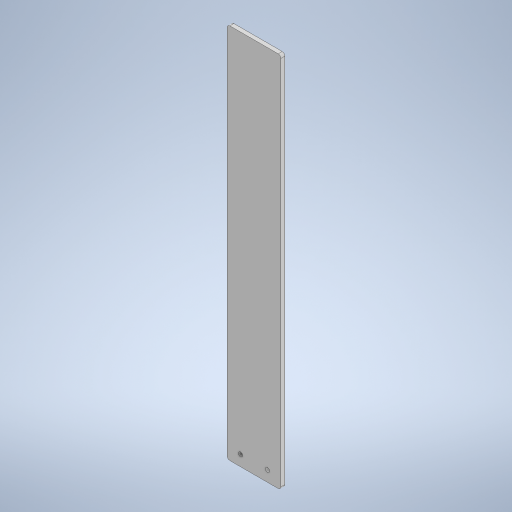
# Autodesk Inventor part: BP_BOX-Support-Bar-Front
Saved by Autodesk Inventor 2024.3 (Build 283343000, 343)
## iProperties
Created: 2025-12-10
Part Number: BP_BOX-Support-Bar-Front
Material: 一般
Document SubType Name: Modeling
Designer: 佐藤智貴
Density: 1 g/cm^3
Appearance: 既定
Author: 佐藤智貴
Autodesk Inventor part; units mm, degrees
ref_plane "YZ Plane" through (0, 0, 0) normal (1, 0, 0) x (0, 1, 0)
ref_plane "XZ Plane" through (0, 0, 0) normal (0, 1, 0) x (-1, 0, 0)
ref_plane "XY Plane" through (0, 0, 0) normal (0, 0, 1) x (1, 0, 0)
sketch "スケッチ1" plane through (0, 0, 0) normal (0, 0, 1) x (1, 0, 0)
  line L0 (0, 0) -> (40, 0)
  line L1 (40, 0) -> (40, 280)
  line L2 (40, 280) -> (0, 280)
  line L3 (0, 280) -> (0, 0)
  dimension "d0" = 40
  dimension "d1" = 280
  constraints: 8 end point, 2 parallel, 1 horizontal, 1 perpendicular
  measures "d0" distance of L1.end L2.end
  measures "d1" distance of L0.end L1.end
extrude "押し出し1" add sketch "スケッチ1" along normal blind 3
sketch "スケッチ2" plane through (0, 0, 3) normal (0, 0, 1) x (1, 0, 0)
  line L0 (0, 280) -> (0, 0) projected
  line L1 (0, 0) -> (40, 0) projected
  point P0 (10, 8)
  point P1 (30, 8)
  point P2 (20, 0)
  dimension "d4" = 20
  dimension "d5" = 10
  dimension "d6" = 8
  constraints: 1 midpoint
  measures "d4" distance of point (30, 8) point (10, 8)
  measures "d5" distance from line of L0 point (10, 8)
  measures "d6" vertical distance of point (10, 8) point (20, 0)
hole "穴1" at (10, 8, 3) at (30, 8, 3) direction (0, 0, -1) diameter 3.2 end through all
fillet "フィレット1" radius 2 4 edges at (0, 0, 1.5) (40, 0, 1.5) (0, 280, 1.5) (40, 280, 1.5)
